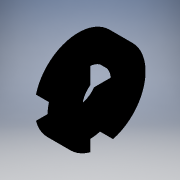
# Autodesk Inventor part: MCOC_spacer26
Saved by Autodesk Inventor 2017.3 (Build 213256000, 256)
## iProperties
Part Number: MCOC_spacer26
Material: Generic
Catalog Web Link: www.cadenas.de
Description: MCOC  Spacer-Couplings - Spacers
Vendor: MISUMI
Document SubType Name: Modeling
Designer: partserver
Manufacturer: MISUMI
Mass: 2.44487 g
Surface Area: 18.2948 cm^2
Volume: 2.44487 cm^3
Density: 1 g/cm^3
Appearance: PSOLRGB-0-0-0
Category: PARTsolutions
Company: MISUMI
Title: MCOC_spacer26
Author: Cadenas PARTsolutions
Comments: Couplings - Spacers
PSOL_IDENT_0: {$CADENAS_DATA\23d-libs\misumi\metric\50_couplings\mcoc\mcoc_spacer.prj},172 {VTYP=3D},{NB=MCOC_spac
PSOL_IDENT_1: er26},{LINA=MCOC_spacer26},{NN=MCOC  Spacer},{DATE=30.03.2018 07:24:20},{GEOMDATE=22.08.2008 00:00:0
PSOL_IDENT_2: 0},{VERSION=},{LINEID=80},{WBVAR=},{WBNUMERIC=}  {NB=MCOC_spacer26},{LINA=MCOC_spacer26},{KT=DUMMY},
PSOL_IDENT_3: {PN=MCOC_spacer26},{MAT=Carbon Reinforced Resin},{TYPE=MCOC_spacer},{NO=26},{D1=27.0},{T=7.2},{DD3=1
PSOL_IDENT_4: 2.0},{W=7.0},{G=4.0},{Z=7.155},{Z1=1.500}
NB: MCOC_spacer26
NN: MCOC  Spacer
NT: Couplings - Spacers
NBSYN: $PN.
LINA: MCOC_spacer26
CATALOG: Misumi
PN: MCOC_spacer26
MAT: Carbon Reinforced Resin
TYPE: MCOC_spacer
NO: 26
D1: 27
T: 7.2
DD3: 12
W: 7
G: 4
Z: 7.155
Z1: 1.5
SUPPLIER: MISUMI
ARTICLENO: MCOC_spacer26
BOMINFO: MCOC_spacer26
CREATOR: CADENAS GmbH
Autodesk Inventor part; units mm, degrees
sketch "Sketch_1" plane through (0, 0, 0) normal (0, 0, 1) x (1, 0, 0)
  line L0 (7.2, 0) -> (0, 0)
  line L1 (0, 6) -> (7.2, 6)
  line L2 (7.2, 6) -> (7.2, 13.5)
  line L3 (7.2, 13.5) -> (0, 13.5)
  line L4 (0, 13.5) -> (0, 6)
  constraints: 10 end point
revolve "Revolution1" add sketch "Sketch_1" angle 360 about axis through (7.2, 0, 0) along (1, 0, 0)
sketch "Sketch_2" plane through (0, 0, 0) normal (0, 0, 1) x (1, 0, 0)
  line L0 (0, 3.5) -> (0, -3.5)
  line L1 (0, -3.5) -> (4, -3.5)
  line L2 (4, -3.5) -> (4, 3.5)
  line L3 (4, 3.5) -> (0, 3.5)
  constraints: 8 end point
extrude "Extrusion1" cut sketch "Sketch_2" along normal mid plane 27
sketch "Sketch_3" plane through (0, 0, 0) normal (0, 1, 0) x (-1, 0, 0)
  line L0 (-3.2, 3.5) -> (-7.2, 3.5)
  line L1 (-7.2, 3.5) -> (-7.2, -3.5)
  line L2 (-7.2, -3.5) -> (-3.2, -3.5)
  line L3 (-3.2, -3.5) -> (-3.2, 3.5)
  constraints: 8 end point
extrude "Extrusion2" cut sketch "Sketch_3" along normal mid plane 27
ref_plane "C_XY" through (3.6, 0, 0) normal (1, 0, 0) x (0, 0, -1)
ref_plane "C_YZ" through (3.6, 0, 0) normal (0, 0, -1) x (0, 1, 0)
ref_plane "C_ZX" through (3.6, 0, 0) normal (0, 1, 0) x (1, 0, 0)
body "Solid1"
